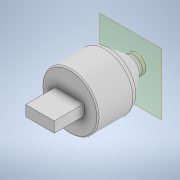
# Autodesk Inventor part: MainHousing_DataPlug
Saved by Autodesk Inventor 2021 (Build 250183000, 183)
## iProperties
Created: 2021-05-07
Part Number: MainHousing_DataPlug
Material: Generic
Document SubType Name: Modeling
Designer: trent
Density: 1 g/cm^3
Appearance: Default
Author: trent
Autodesk Inventor part; units mm, degrees
ref_plane "YZ Plane" through (0, 0, 0) normal (1, 0, 0) x (0, 1, 0)
ref_plane "XZ Plane" through (0, 0, 0) normal (0, 1, 0) x (-1, 0, 0)
ref_plane "XY Plane" through (0, 0, 0) normal (0, 0, 1) x (1, 0, 0)
sketch "Sketch1" plane through (0, 0, 0) normal (0, 0, 1) x (1, 0, 0)
  circle A0 centre (0, 0) radius 12
  line L0 (-6.1, 2.275) -> (6.1, 2.275)
  line L1 (6.1, 2.275) -> (6.1, -2.275)
  line L2 (6.1, -2.275) -> (-6.1, -2.275)
  line L3 (-6.1, -2.275) -> (-6.1, 2.275)
  dimension "d0" = 12.2
  dimension "d1" = 4.55
  dimension "d2" = 2.275
  dimension "d3" = 6.1
  dimension "d4" = 24
  constraints: 8 end point, 2 parallel, 1 centre point, 1 coincident, 1 horizontal, 1 perpendicular
  measures "d0" distance of L0.start L0.end
  measures "d1" distance of L2.end L0.start
  measures "d2" distance from line of point (0, 0) L0
  measures "d3" distance from line of point (0, 0) L3
  measures "d4" diameter of A0
extrude "Extrusion1" add sketch "Sketch1" along normal blind 16
ref_plane "Work Plane1" through (0, 0, -10) normal (0, 0, -1) x (-1, 0, 0)
sketch "Sketch4" plane through (0, 0, -10) normal (0, 0, -1) x (-1, 0, 0)
  circle A0 centre (0, 0) radius 4
  dimension "d11" = 8
  constraints: 1 centre point, 1 coincident
  measures "d11" diameter of A0
extrude "Extrusion3" add sketch "Sketch4" along normal blind 4
sketch "Sketch6" plane through (0, 0, 0) normal (0, 0, -1) x (-1, 0, 0)
  circle A0 centre (0, 0) radius 12
  constraints: 1 centre point, 1 coincident
loft "Loft1" add profiles "Sketch6" section 2 edges at (4, 0, -10)
sketch "Sketch7" plane through (0, 0, -14) normal (0, 0, -1) x (-1, 0, 0)
  circle A0 centre (0, 0) radius 4 projected
  circle A1 centre (0, 0) radius 2
  dimension "d18" = 4
  constraints: 1 centre point, 1 coincident
  measures "d18" diameter of A1
extrude "Extrusion4" cut sketch "Sketch7" against normal blind 6 contours A1
loft "Loft2" cut section 1 edges at (-6.1, 0, 0) (0, -2.275, 0) (6.1, 0, 0) (0, 2.275, 0) section 2 edges at (2, 0, -8)
fillet "Fillet1" radius 1.5 1 edges at (4, 0, -14)
fillet "Fillet2" radius 3 1 edges at (4, 0, -10)
fillet "Fillet3" radius 3 2 edges at (0, 12, 0) (0, -12, 0)
fillet "Fillet4" radius 0.5 1 edges at (-12, 0, 16)
sketch "Sketch8" plane through (0, 0, 16) normal (0, 0, 1) x (1, 0, 0)
  line L0 (-6.1, 2.275) -> (6.1, 2.275) projected
  line L1 (6.1, -2.275) -> (-6.1, -2.275) projected
  line L2 (-6.1, 2.275) -> (6.1, 2.275)
  line L3 (6.1, 2.275) -> (6.1, -2.275)
  line L4 (6.1, -2.275) -> (-6.1, -2.275)
  line L5 (-6.1, -2.275) -> (-6.1, 2.275)
  point P0 (0, 0)
  point P1 (-6.1, -2.275)
  constraints: 8 end point, 2 parallel, 1 horizontal, 1 perpendicular
extrude "Extrusion5" add sketch "Sketch8" along normal blind 12.75
equation "\"d2\" = 0.5 * d1"
equation "\"d3\" = 0.5 * d0"
body "Solid1"
